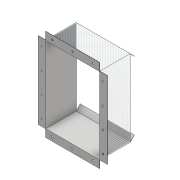
# Autodesk Inventor part: chimneyHousing
Saved by Autodesk Inventor 2017 (Build 210142000, 142)
## iProperties
Created: 2016-12-02
Part Number: chimneyHousing
Material: Generic
Document SubType Name: Modeling
Designer: krosie
Density: 1 g/cm^3
Appearance: Default
Author: krosie
Autodesk Inventor part; units mm, degrees
ref_plane "YZ Plane" through (0, 0, 0) normal (1, 0, 0) x (0, 1, 0)
ref_plane "XZ Plane" through (0, 0, 0) normal (0, 1, 0) x (-1, 0, 0)
ref_plane "XY Plane" through (0, 0, 0) normal (0, 0, 1) x (1, 0, 0)
sketch "Sketch1" plane through (0, 0, 0) normal (0, 1, 0) x (-1, 0, 0)
  line L0 (-89, 127) -> (89, 127)
  line L1 (89, 127) -> (89, -127)
  line L2 (89, -127) -> (-89, -127)
  line L3 (-89, -127) -> (-89, 127)
  line L4 (-89, 127) -> (89, -127) construction
  line L5 (89, 127) -> (-89, -127) construction
  line L6 (90, 128) -> (-90, 128)
  line L7 (-90, 128) -> (-90, -128)
  line L8 (-90, -128) -> (90, -128)
  line L9 (90, -128) -> (90, 128)
  point P0 (0, 0)
  dimension "d0" = 178
  dimension "d1" = 254
  dimension "d2" = 1
  constraints: 20 end point, 4 parallel, 2 midpoint, 2 perpendicular, 1 horizontal, 3 other
  measures "d0" distance of L1.end L2.end
  measures "d1" distance of L0.end L1.end
  measures "d2" distance between parallel lines of L0 L6
extrude "Extrusion1" add sketch "Sketch1" along normal blind 101.6
sketch "Sketch3" plane through (0, 0, 0) normal (0, -1, 0) x (1, 0, 0)
  line L0 (90, 128) -> (90, -128) projected
  line L1 (90, -128) -> (-90, -128) projected
  line L2 (90, 128) -> (90, -128)
  line L3 (90, -128) -> (115, -128)
  line L4 (115, -128) -> (115, 128)
  line L5 (115, 128) -> (90, 128)
  line L6 (90, -128) -> (-90, -128)
  line L7 (-90, -128) -> (-90, -153)
  line L8 (-90, -153) -> (90, -153)
  line L9 (90, -153) -> (90, -128)
  line L10 (-90, 128) -> (90, 128) projected
  line L11 (-90, -128) -> (-90, 128)
  line L12 (-90, 128) -> (-115, 128)
  line L13 (-115, 128) -> (-115, -128)
  line L14 (-115, -128) -> (-90, -128)
  line L15 (-90, 128) -> (90, 128)
  line L16 (90, 128) -> (90, 153)
  line L17 (90, 153) -> (-90, 153)
  line L18 (-90, 153) -> (-90, 128)
  point P0 (0, 0)
  dimension "d11" = 25
  dimension "d12" = 25
  dimension "d13" = 25
  dimension "d14" = 25
  constraints: 32 end point, 9 parallel, 4 perpendicular, 2 collinear, 1 vertical
  measures "d11" distance of L3.end L0.end
  measures "d12" distance of L7.end L1.end
  measures "d13" distance of L12.end L10.start
  measures "d14" distance of L16.end L0.start
extrude "Extrusion3" add sketch "Sketch3" against normal blind 0.8 contours L5 L4 L3 L0 | L10 L18 L17 L16 | L9 L8 L7 L1 | L11 L14 L13 L12
sketch "Sketch4" plane through (0, 0.8, 0) normal (0, 1, 0) x (1, 0, 0)
  line L0 (101.5, 139.5) -> (-101.5, 139.5) construction
  line L1 (-101.5, 139.5) -> (-101.5, -139.5) construction
  line L2 (-101.5, -139.5) -> (101.5, -139.5) construction
  line L3 (101.5, -139.5) -> (101.5, 139.5) construction
  line L4 (101.5, 139.5) -> (-101.5, -139.5) construction
  line L5 (-101.5, 139.5) -> (101.5, -139.5) construction
  line L6 (0, 0) -> (0, -60) construction
  line L7 (0, 0) -> (60, 0) construction
  point P0 (-101.5, 0)
  point P1 (101.5, 0)
  point P2 (101.5, 104.625)
  point P3 (101.5, 69.75)
  point P4 (101.5, 34.875)
  point P5 (101.5, 0)
  point P6 (101.5, -34.875)
  point P7 (101.5, -69.75)
  point P8 (101.5, -104.625)
  point P9 (67.6667, 139.5)
  point P10 (33.8333, 139.5)
  point P11 (0, 139.5)
  point P12 (-33.8333, 139.5)
  point P13 (-67.6667, 139.5)
  point P14 (-101.5, 139.5)
  point P15 (67.6667, -139.5)
  point P16 (33.8333, -139.5)
  point P17 (0, -139.5)
  point P18 (-33.8333, -139.5)
  point P19 (-67.6667, -139.5)
  point P20 (-101.5, -139.5)
  point P21 (-101.5, 104.625)
  point P22 (-101.5, 69.75)
  point P23 (-101.5, 34.875)
  point P24 (-101.5, 0)
  point P25 (-101.5, -34.875)
  point P26 (-101.5, -69.75)
  point P27 (-101.5, -104.625)
  dimension "d18" = 203
  dimension "d19" = 279
  dimension "d21" = 60
  dimension "d22" = 90
  dimension "d63" = 34.875
  dimension "d70" = 33.8333
  dimension "d77" = 33.8333
  dimension "d84" = 34.875
  constraints: 16 end point, 4 horizontal, 4 midpoint, 3 vertical, 2 parallel, 2 perpendicular, 1 coincident, 27 other
  measures "d18" distance of L2.end L1.end
  measures "d19" distance of L1.end L0.end
  measures "d21" distance of L6.start L6.end
  measures "d22" angle of L6 L7
  measures "d63" distance of point (101.5, 139.5) point (101.5, 104.625)
  measures "d70" distance of point (101.5, 139.5) point (67.667, 139.5)
  measures "d77" distance of point (101.5, -139.5) point (67.667, -139.5)
  measures "d84" distance of point (-101.5, 139.5) point (-101.5, 104.625)
hole "Hole1" at (101.5, 0.8, -139.5) at (101.5, 0.8, -104.625) at (101.5, 0.8, -34.875) at (101.5, 0.8, 34.875) at (101.5, 0.8, 104.625) at (101.5, 0.8, 139.5) at (67.6667, 0.8, -139.5) at (0, 0.8, -139.5) at (-67.6667, 0.8, -139.5) at (-101.5, 0.8, -139.5) at (67.6667, 0.8, 139.5) at (0, 0.8, 139.5) at (-67.6667, 0.8, 139.5) at (-101.5, 0.8, 139.5) at (-101.5, 0.8, -104.625) at (-101.5, 0.8, -34.875) at (-101.5, 0.8, 34.875) at (-101.5, 0.8, 104.625) direction (0, -1, 0) diameter 6 end through all
sketch "Sketch9" plane through (90, 0.8, 128) normal (1, 0, 0) x (0, 0, -1)
  line L0 (0, 100.8) -> (14.1421, 114.9421)
  line L1 (0, 100.8) -> (20, 100.8) construction
  line L2 (14.5421, 114.5421) -> (0.8, 100.8)
  line L3 (14.1421, 114.9421) -> (14.5421, 114.5421)
  line L4 (256, 0) -> (256, 100.8) projected
  line L5 (256, 100.8) -> (241.8579, 114.9421)
  line L6 (256, 100.8) -> (276, 100.8) construction
  line L7 (0, 100.8) -> (256, 100.8) projected
  line L8 (229, 100.8) -> (256, 100.8)
  line L9 (256, 100.8) -> (0, 100.8) projected
  line L10 (0, 100.8) -> (0.8, 100.8)
  line L11 (241.2922, 114.3765) -> (254.8686, 100.8)
  line L12 (241.8579, 114.9421) -> (241.2922, 114.3765)
  point P0 (128, -0.8)
  dimension "d51" = 20
  dimension "d52" = 45
  dimension "d53" = 20
  dimension "d54" = 135
  dimension "d89" = 0.8
  constraints: 20 end point, 3 point on line, 2 collinear, 2 equal length, 2 horizontal, 2 perpendicular, 1 coincident, 1 parallel
  measures "d51" distance of L0.start L0.end
  measures "d52" angle of L1 L0
  measures "d53" distance of L4.end L5.end
  measures "d54" angle of L6 L5
  measures "d89" distance between parallel lines of L5 L11
extrude "Extrusion8" add sketch "Sketch9" against normal up to surface (180 mm away)
body "Solid1"
